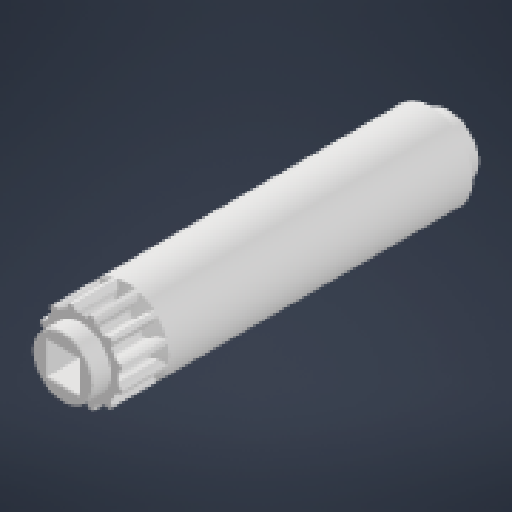
# Autodesk Inventor part: Bio12tNew
Saved by Autodesk Inventor 2024.1 (Build 281209000, 209)
## iProperties
Created: 2023-11-14
Part Number: Bio12tNew
Material: Generic
Document SubType Name: Modeling
Designer: Brandon
Density: 1 g/cm^3
Appearance: Default
Author: Brandon
Autodesk Inventor part; units mm, degrees
ref_plane "YZ Plane" through (0, 0, 0) normal (1, 0, 0) x (0, 1, 0)
ref_plane "XZ Plane" through (0, 0, 0) normal (0, 1, 0) x (-1, 0, 0)
ref_plane "XY Plane" through (0, 0, 0) normal (0, 0, 1) x (1, 0, 0)
sketch "Sketch1" plane through (0, 0, 0) normal (0, 0, 1) x (1, 0, 0)
  spline S0 degree 3 poles (-1.1349, 5.2119) (-1.1074, 5.185) (-1.0524, 5.1313) (-0.9744, 5.0464) (-0.8999, 4.9583) (-0.8297, 4.8668) (-0.7645, 4.7717) (-0.7049, 4.6729) (-0.6613, 4.5872) (-0.6305, 4.5167) (-0.6177, 4.4805) (-0.6113, 4.4624) knots 0 0 0 0 0.125004 0.250011 0.375016 0.50002 0.62502 0.750015 0.875 0.937503 1 1 1 1
  spline S1 degree 3 poles (-0.6113, 4.4624) (-0.6155, 4.4339) (-0.624, 4.3769) (-0.6308, 4.2907) (-0.6327, 4.2043) (-0.6308, 4.1179) (-0.622, 4.0319) (-0.6073, 3.9467) (-0.5851, 3.8631) (-0.5552, 3.7819) (-0.5159, 3.7048) (-0.4749, 3.6453) (-0.4366, 3.6023) (-0.4054, 3.5723) (-0.3718, 3.5452) (-0.3356, 3.5214) (-0.2974, 3.5013) (-0.2572, 3.4852) (-0.2154, 3.4739) (-0.1727, 3.4669) (-0.1295, 3.4646) (-0.072, 3.4669) (0, 3.4676) (0.072, 3.4669) (0.1295, 3.4646) (0.1727, 3.4669) (0.2154, 3.4739) (0.2572, 3.4852) (0.2974, 3.5013) (0.3356, 3.5214) (0.3718, 3.5452) (0.4054, 3.5723) (0.4366, 3.6023) (0.4749, 3.6453) (0.5159, 3.7048) (0.5552, 3.7819) (0.5851, 3.8631) (0.6073, 3.9467) (0.622, 4.0319) (0.6308, 4.1179) (0.6327, 4.2043) (0.6308, 4.2907) (0.624, 4.3769) (0.6155, 4.4339) (0.6113, 4.4624) knots 0 0 0 0 0.031253 0.062508 0.093762 0.125013 0.156265 0.187519 0.218767 0.250016 0.281263 0.312504 0.328134 0.343755 0.359376 0.375 0.390627 0.406258 0.421885 0.4375 0.453117 0.468749 0.5 0.531251 0.546883 0.5625 0.578115 0.593742 0.609373 0.625 0.640624 0.656245 0.671866 0.687496 0.718737 0.749984 0.781233 0.812481 0.843735 0.874987 0.906238 0.937492 0.968747 1 1 1 1
  spline S2 degree 3 poles (0.6113, 4.4624) (0.6177, 4.4805) (0.6305, 4.5167) (0.6613, 4.5872) (0.7049, 4.6729) (0.7645, 4.7717) (0.8297, 4.8668) (0.8999, 4.9583) (0.9744, 5.0464) (1.0524, 5.1313) (1.1074, 5.185) (1.1349, 5.2119) knots 0 0 0 0 0.062497 0.125 0.249985 0.37498 0.49998 0.624984 0.749989 0.874996 1 1 1 1
  circle A0 centre (0, 0) radius 3.4673 construction
  circle A1 centre (0, 0) radius 4.4264 construction
  circle A2 centre (0, 0) radius 4.572 construction
  circle A3 centre (0, 0) radius 5.334
  point P0 (-1.0532, 5.1306)
  point P1 (-0.975, 5.0458)
  point P2 (-0.9006, 4.9577)
  point P3 (-0.8305, 4.8662)
  point P4 (-0.7654, 4.771)
  point P5 (-0.7061, 4.6722)
  point P6 (-0.6539, 4.5694)
  point P7 (-0.6311, 4.5165)
  point P8 (-0.623, 4.3768)
  point P9 (-0.63, 4.2907)
  point P10 (-0.632, 4.2043)
  point P11 (-0.6297, 4.118)
  point P12 (-0.621, 4.0321)
  point P13 (-0.6061, 3.947)
  point P14 (-0.5838, 3.8635)
  point P15 (-0.5537, 3.7826)
  point P16 (-0.5143, 3.7058)
  point P17 (-0.4649, 3.6349)
  point P18 (-0.4362, 3.6027)
  point P19 (-0.405, 3.5728)
  point P20 (-0.3714, 3.5457)
  point P21 (-0.3353, 3.522)
  point P22 (-0.297, 3.502)
  point P23 (-0.2569, 3.486)
  point P24 (-0.2152, 3.4746)
  point P25 (-0.1726, 3.4677)
  point P26 (-0.1296, 3.4653)
  point P27 (-0.0864, 3.4662)
  point P28 (0, 3.4673)
  point P29 (0.0864, 3.4662)
  point P30 (0.1296, 3.4653)
  point P31 (0.1726, 3.4677)
  point P32 (0.2152, 3.4746)
  point P33 (0.2569, 3.486)
  point P34 (0.297, 3.502)
  point P35 (0.3353, 3.522)
  point P36 (0.3714, 3.5457)
  point P37 (0.405, 3.5728)
  point P38 (0.4362, 3.6027)
  point P39 (0.4649, 3.6349)
  point P40 (0.5143, 3.7058)
  point P41 (0.5537, 3.7826)
  point P42 (0.5838, 3.8635)
  point P43 (0.6061, 3.947)
  point P44 (0.621, 4.0321)
  point P45 (0.6297, 4.118)
  point P46 (0.632, 4.2043)
  point P47 (0.63, 4.2907)
  point P48 (0.623, 4.3768)
  point P49 (0.6311, 4.5165)
  point P50 (0.6539, 4.5694)
  point P51 (0.7061, 4.6722)
  point P52 (0.7654, 4.771)
  point P53 (0.8305, 4.8662)
  point P54 (0.9006, 4.9577)
  point P55 (0.975, 5.0458)
  point P56 (1.0532, 5.1306)
  constraints: 4 centre point, 2 point on circle, 129 other
extrude "Extrusion1" add sketch "Sketch1" against normal blind 18.542
extrude "Extrusion2" cut sketch "Sketch1" against normal through all contours A3 S2 S1 S0 picked at (0.127, 4.7484)
pattern_circular "Circular Pattern1" count 12 over 360 about axis through (0, 0, 0) along (0, 0, -1) of "Extrusion2"
sketch "Sketch2" plane through (0, 0, 0) normal (0, 0, 1) x (1, 0, 0)
  arc A0 (-3.5888, 3.9462) -> (-3.9462, 3.5888) centre (0, 0) ccw projected
  arc A1 (-5.0811, 1.6231) -> (-5.2119, 1.1349) centre (0, 0) ccw projected
  arc A2 (-5.2119, -1.1349) -> (-5.0811, -1.6231) centre (0, 0) ccw projected
  arc A3 (-3.9462, -3.5888) -> (-3.5888, -3.9462) centre (0, 0) ccw projected
  arc A4 (-1.6231, -5.0811) -> (-1.1349, -5.2119) centre (0, 0) ccw projected
  arc A5 (1.1349, -5.2119) -> (1.6231, -5.0811) centre (0, 0) ccw projected
  arc A6 (3.5888, -3.9462) -> (3.9462, -3.5888) centre (0, 0) ccw projected
  arc A7 (5.0811, -1.6231) -> (5.2119, -1.1349) centre (0, 0) ccw projected
  arc A8 (5.2119, 1.1349) -> (5.0811, 1.6231) centre (0, 0) ccw projected
  arc A9 (3.9462, 3.5888) -> (3.5888, 3.9462) centre (0, 0) ccw projected
  arc A10 (1.6231, 5.0811) -> (1.1349, 5.2119) centre (0, 0) ccw projected
  arc A11 (-1.1349, 5.2119) -> (-1.6231, 5.0811) centre (0, 0) ccw projected
  circle A12 centre (0, 0) radius 3.175
  line L0 (-2.032, 2.032) -> (2.032, 2.032)
  line L1 (2.032, 2.032) -> (2.032, -2.032)
  line L2 (2.032, -2.032) -> (-2.032, -2.032)
  line L3 (-2.032, -2.032) -> (-2.032, 2.032)
  line L4 (-2.032, 2.032) -> (2.032, -2.032) construction
  line L5 (2.032, 2.032) -> (-2.032, -2.032) construction
  dimension "d7" = 6.35
  dimension "d8" = 4.064
  dimension "d9" = 4.064
  constraints: 12 end point, 2 horizontal alignment, 2 midpoint, 2 parallel, 2 vertical alignment, 1 centre point, 1 coincident, 1 horizontal, 1 perpendicular, 32 other
  measures "d7" diameter of A12
  measures "d8" distance of L1.end L2.end
  measures "d9" distance of L0.end L1.end
extrude "Extrusion3" add sketch "Sketch2" along normal blind 2.0955
extrude "Extrusion4" cut sketch "Sketch2" against normal blind 4.7625 contours L0 L1 L2 L3
chamfer "Chamfer1" distance 0.127 angle 45 4 edges at (0, 2.032, 2.0955) (-2.032, 0, 2.0955) (2.032, 0, 2.0955) (0, -2.032, 2.0955)
sketch "Sketch3" plane through (0, 0, 0) normal (1, 0, 0) x (0, 1, 0)
  line L0 (3.7361, -0.762) -> (1.6285, -0.762) projected
  line L1 (3.5714, -4.572) -> (5.6026, -4.572) projected
  line L2 (5.6026, -0.762) -> (3.5714, -0.762) projected
  line L3 (-3.175, 0) -> (3.175, 0) projected
  line L4 (3.175, 0) -> (3.175, 2.0955) projected
  line L5 (3.175, 0) -> (3.175, -0.762)
  line L6 (4.4624, -18.542) -> (4.4624, -18.542) projected
  line L7 (4.4624, 0) -> (4.4624, -18.542) projected
  line L8 (4.4624, 0) -> (4.4624, 0) projected
  line L9 (4.4624, 0) -> (4.4624, -18.542) projected
  line L10 (3.447, -0.762) -> (4.7668, 0)
  line L11 (4.7668, 0) -> (3.175, 0)
  line L12 (0, -22.7227) -> (0, 6.5282) projected
  line L13 (0, -2.6325) -> (5.334, -5.7121)
  line L14 (3.175, 0) -> (5.334, 0)
  line L15 (5.334, 0) -> (5.334, -5.7121)
  line L16 (5.334, -5.7121) -> (3.0759, -5.7121)
  line L17 (3.0759, -5.7121) -> (3.2928, -4.4179)
  point P0 (0, 0)
  point P1 (3.175, 2.2225)
  point P2 (-3.175, 2.2225)
  point P3 (3.2751, -4.5234)
  dimension "d17" = 30
  dimension "d19" = 30
  dimension "d20" = 2.159
  constraints: 16 end point, 4 point on line, 2 horizontal, 2 perpendicular, 1 horizontal alignment, 1 other
  measures "d17" angle of L2 L10
  measures "d19" angle of L1 L13
  measures "d20" distance of L4.start L14.end
revolve "Revolution1" add sketch "Sketch3" angle 360 about axis through (0, 0, -10) along (0, 0, 1) contours L0 L5 L11 L7 L10 | L7 L11 L10
revolve "Revolution2" add sketch "Sketch3" angle 360 about axis through (0, 0, -10) along (0, 0, 1) contours L13 L16 L7 | L7 L16 L17 L13
sketch "Sketch4" plane through (0, 0, -18.542) normal (0, 0, -1) x (-1, 0, 0)
  arc A0 (-1.6231, 5.0811) -> (-3.5888, 3.9462) centre (0, 0) ccw projected
  circle A1 centre (0, 0) radius 5.334
  point P0 (-3.5888, 3.9462)
  constraints: 1 coincident, 3 other
extrude "Extrusion5" add sketch "Sketch4" along normal blind 25.5397 and the other way blind 12.8299
sketch "Sketch5" plane through (0, 0, 0) normal (0, 0, 1) x (1, 0, 0)
  circle A0 centre (0, 0) radius 3.175 projected
  arc A1 (-1.1349, 5.2119) -> (-1.6231, 5.0811) centre (0, 0) ccw projected
  arc A2 (-1.7247, 4.4438) -> (-2.9861, 3.7156) centre (0, 0) ccw projected
  arc A3 (-3.5888, 3.9462) -> (-3.9462, 3.5888) centre (0, 0) ccw projected
  arc A4 (-3.7156, 2.9861) -> (-4.4438, 1.7247) centre (0, 0) ccw projected
  arc A5 (-5.0811, 1.6231) -> (-5.2119, 1.1349) centre (0, 0) ccw projected
  arc A6 (-4.7108, 0.7283) -> (-4.7108, -0.7283) centre (0, 0) ccw projected
  arc A7 (-5.2119, -1.1349) -> (-5.0811, -1.6231) centre (0, 0) ccw projected
  arc A8 (-4.4438, -1.7247) -> (-3.7156, -2.9861) centre (0, 0) ccw projected
  arc A9 (-3.9462, -3.5888) -> (-3.5888, -3.9462) centre (0, 0) ccw projected
  arc A10 (-2.9861, -3.7156) -> (-1.7247, -4.4438) centre (0, 0) ccw projected
  arc A11 (-1.6231, -5.0811) -> (-1.1349, -5.2119) centre (0, 0) ccw projected
  arc A12 (-0.7283, -4.7108) -> (0.7283, -4.7108) centre (0, 0) ccw projected
  arc A13 (1.1349, -5.2119) -> (1.6231, -5.0811) centre (0, 0) ccw projected
  arc A14 (1.7247, -4.4438) -> (2.9861, -3.7156) centre (0, 0) ccw projected
  arc A15 (3.5888, -3.9462) -> (3.9462, -3.5888) centre (0, 0) ccw projected
  arc A16 (3.7156, -2.9861) -> (4.4438, -1.7247) centre (0, 0) ccw projected
  arc A17 (5.0811, -1.6231) -> (5.2119, -1.1349) centre (0, 0) ccw projected
  arc A18 (4.7108, -0.7283) -> (4.7108, 0.7283) centre (0, 0) ccw projected
  arc A19 (5.2119, 1.1349) -> (5.0811, 1.6231) centre (0, 0) ccw projected
  arc A20 (4.4438, 1.7247) -> (3.7156, 2.9861) centre (0, 0) ccw projected
  arc A21 (3.9462, 3.5888) -> (3.5888, 3.9462) centre (0, 0) ccw projected
  arc A22 (2.9861, 3.7156) -> (1.7247, 4.4438) centre (0, 0) ccw projected
  arc A23 (1.6231, 5.0811) -> (1.1349, 5.2119) centre (0, 0) ccw projected
  arc A24 (0.7283, 4.7108) -> (-0.7283, 4.7108) centre (0, 0) ccw projected
  circle A25 centre (0, 0) radius 3.81
  dimension "d26" = 7.62
  constraints: 1 centre point, 1 coincident, 24 other
  measures "d26" diameter of A25
extrude "Extrusion6" add sketch "Sketch5" along normal up to surface (2.0955 mm away)
chamfer "Chamfer2" distance 0.127 angle 45 1 edges at (-3.81, 0, 2.0955)
sketch "Sketch6" plane through (0, 0, -44.0817) normal (0, 0, -1) x (-1, 0, 0)
  circle A0 centre (0, 0) radius 3.81 projected
  arc A1 (1.6231, 5.0811) -> (1.1349, 5.2119) centre (0, 0) ccw projected
  arc A2 (2.9861, 3.7156) -> (1.7247, 4.4438) centre (0, 0) ccw projected
  arc A3 (3.9462, 3.5888) -> (3.5888, 3.9462) centre (0, 0) ccw projected
  arc A4 (4.4438, 1.7247) -> (3.7156, 2.9861) centre (0, 0) ccw projected
  arc A5 (5.2119, 1.1349) -> (5.0811, 1.6231) centre (0, 0) ccw projected
  arc A6 (4.7108, -0.7283) -> (4.7108, 0.7283) centre (0, 0) ccw projected
  arc A7 (5.0811, -1.6231) -> (5.2119, -1.1349) centre (0, 0) ccw projected
  arc A8 (3.7156, -2.9861) -> (4.4438, -1.7247) centre (0, 0) ccw projected
  arc A9 (3.5888, -3.9462) -> (3.9462, -3.5888) centre (0, 0) ccw projected
  arc A10 (1.7247, -4.4438) -> (2.9861, -3.7156) centre (0, 0) ccw projected
  arc A11 (1.1349, -5.2119) -> (1.6231, -5.0811) centre (0, 0) ccw projected
  arc A12 (-0.7283, -4.7108) -> (0.7283, -4.7108) centre (0, 0) ccw projected
  arc A13 (-1.6231, -5.0811) -> (-1.1349, -5.2119) centre (0, 0) ccw projected
  arc A14 (-2.9861, -3.7156) -> (-1.7247, -4.4438) centre (0, 0) ccw projected
  arc A15 (-3.9462, -3.5888) -> (-3.5888, -3.9462) centre (0, 0) ccw projected
  arc A16 (-4.4438, -1.7247) -> (-3.7156, -2.9861) centre (0, 0) ccw projected
  arc A17 (-5.2119, -1.1349) -> (-5.0811, -1.6231) centre (0, 0) ccw projected
  arc A18 (-4.7108, 0.7283) -> (-4.7108, -0.7283) centre (0, 0) ccw projected
  arc A19 (-5.0811, 1.6231) -> (-5.2119, 1.1349) centre (0, 0) ccw projected
  arc A20 (-3.7156, 2.9861) -> (-4.4438, 1.7247) centre (0, 0) ccw projected
  arc A21 (-3.5888, 3.9462) -> (-3.9462, 3.5888) centre (0, 0) ccw projected
  arc A22 (-1.7247, 4.4438) -> (-2.9861, 3.7156) centre (0, 0) ccw projected
  arc A23 (-1.1349, 5.2119) -> (-1.6231, 5.0811) centre (0, 0) ccw projected
  arc A24 (0.7283, 4.7108) -> (-0.7283, 4.7108) centre (0, 0) ccw projected
  line L0 (-2.032, -2.032) -> (2.032, -2.032) projected
  line L1 (-2.032, 2.032) -> (-2.032, -2.032) projected
  line L2 (2.032, 2.032) -> (-2.032, 2.032) projected
  line L3 (2.032, -2.032) -> (2.032, 2.032) projected
  constraints: 24 other
extrude "Extrusion7" add sketch "Sketch6" along normal blind 2.3495
chamfer "Chamfer3" distance 0.127 angle 45 5 edges at (3.81, 0, -46.4312) (-2.032, 0, -46.4312) (0, 2.032, -46.4312) (2.032, 0, -46.4312) (0, -2.032, -46.4312)
extrude "Extrusion8" cut sketch "Sketch6" against normal blind 4.7625 contours L1 L2 L3 L0
sketch "Sketch7" plane through (0, 0, -4.7625) normal (0, 0, 1) x (1, 0, 0)
  circle A0 centre (0, 0) radius 1.524
  dimension "d39" = 3.048
  constraints: 1 centre point, 1 coincident
  measures "d39" diameter of A0
extrude "Extrusion9" cut sketch "Sketch7" against normal blind 4.2545
chamfer "Chamfer4" distance 0.127 angle 45 1 edges at (-1.524, 0, -4.7625)
equation "\"d0\" = FaceWidth"
equation "\"Module\" = 0.762"
equation "\"PressureAngle\" = 14.5deg"
equation "\"UnitProfileClearance\" = 0.25"
equation "\"UnitRoundRadius\" = 0.3335"
equation "\"HeadDiameter\" = 10.668"
equation "\"RootDiameter\" = 6.93466"
equation "\"BaseDiameter\" = 8.85274"
equation "\"PitchDiameter\" = 9.144"
equation "\"FaceWidth\" = 18.542"
equation "\"HelixAngle\" = 0"
equation "\"UnitCorrection\" = 0"
equation "\"UnitAddendumModification\" = 0"
equation "\"CircularPitch\" = 2.39389"
equation "\"UnitBacklashShift\" = -0.199696"
equation "\"TotalToolShift\" = -0.15217"
equation "\"IsInternal\" = 0"
body "Solid1"
